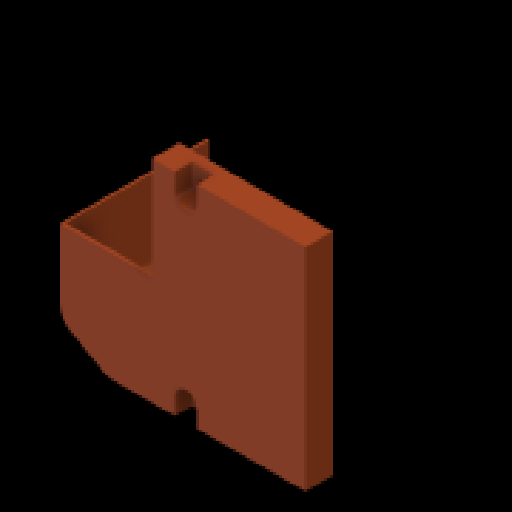
# Autodesk Inventor part: Extruder Cover
Saved by Autodesk Inventor 2023.3 (Build 273359000, 359)
## iProperties
Created: 2023-02-08
Part Number: Extruder Cover
Material: ABS Plastic
Document SubType Name: Modeling
Designer: remop
Density: 1.06 g/cm^3
Appearance: Smooth - Light Orange
Author: remop
Autodesk Inventor part; units mm, degrees
ref_plane "YZ Plane" through (0, 0, 0) normal (1, 0, 0) x (0, 1, 0)
ref_plane "XZ Plane" through (0, 0, 0) normal (0, 1, 0) x (-1, 0, 0)
ref_plane "XY Plane" through (0, 0, 0) normal (0, 0, 1) x (1, 0, 0)
sketch "Sketch1" plane through (0, 0, 0) normal (0, 0, 1) x (1, 0, 0)
  circle A0 centre (-5, 44) radius 1.4 projected
  circle A1 centre (-5, -8) radius 1.4 projected
  circle A2 centre (-5, 44) radius 1.75
  circle A3 centre (-5, -8) radius 1.75
  circle A4 centre (-5, -8) radius 3.25
  line L0 (-10, 49) -> (30, 49) projected
  line L1 (-10, -13) -> (30, -13) projected
  circle A5 centre (-5, 44) radius 3.25
  line L2 (-1.75, 44) -> (-1.75, 49)
  line L3 (-1.75, -8) -> (-1.75, -13)
  line L4 (-8.25, 44) -> (-8.25, 49)
  line L5 (-8.25, -8) -> (-8.25, -13)
  line L6 (-39, 42.6491) -> (-29.3923, 48.1962) projected
  arc A6 (-39, 42.6491) -> (-42, 37.453) centre (-36, 37.453) ccw projected
  line L7 (-42, -1.453) -> (-42, 37.453) projected
  arc A7 (-42, -1.453) -> (-39, -6.6491) centre (-36, -1.453) ccw projected
  line L8 (-39, -6.6491) -> (-29.3923, -12.1962) projected
  arc A8 (-29.3923, -12.1962) -> (-26.3923, -13) centre (-26.3923, -7) ccw projected
  line L9 (-26.3923, -13) -> (-21.4462, -13) projected
  arc A9 (-26.3923, 49) -> (-29.3923, 48.1962) centre (-26.3923, 43) ccw projected
  line L10 (-10, 49) -> (-38, 49) projected
  line L11 (-10, -13) -> (-21.4462, -13)
  line L12 (30, 49) -> (30, -13)
  circle A10 centre (-26.3923, -7) radius 6
  circle A11 centre (-36, -1.453) radius 6
  circle A12 centre (-36, 37.453) radius 6
  circle A13 centre (-26.3923, 43) radius 6
  line L13 (-29.3923, 48.1962) -> (-39, 42.6491)
  line L14 (-42, 37.453) -> (-42, -1.453)
  line L15 (-39, -6.6491) -> (-29.3923, -12.1962)
  line L16 (-26.3923, -13) -> (-8.25, -13)
  line L17 (-1.75, -13) -> (30, -13)
  line L18 (30, 49) -> (-1.75, 49)
  line L19 (-8.25, 49) -> (-26.3923, 49)
  point P0 (0, 0)
  dimension "d0" = 3.5
  dimension "d1" = 6.5
  constraints: 26 end point, 11 point on line, 8 coincident, 6 point on circle, 5 centre point, 5 tangent, 4 collinear, 4 vertical, 2 equal radius, 1 horizontal, 1 perpendicular, 1 vertical alignment, 11 other
  measures "d0" diameter of A3
  measures "d1" diameter of A4
extrude "Extrusion1" add sketch "Sketch1" along normal blind 7 contours A4 L5 L1 L11 L9 A10 A11 L7 A12 A13 L10 L0 L4 A5 L2 L12 L3 | A8 A10 A11 | L8 A11 A10 | A7 A11 A10 | A10 A11 | A13 A12 A9 | A13 A12 L6 | A6 A12 A13 | A12 A13
sketch "Sketch2" plane through (0, 0, 7) normal (0, 0, 1) x (1, 0, 0)
  line L0 (30, 49) -> (-1.75, 49) projected
  line L1 (-1.75, 49) -> (-1.75, 44) projected
  arc A0 (-8.25, 44) -> (-1.75, 44) centre (-5, 44) ccw projected
  line L2 (-8.25, 44) -> (-8.25, 49) projected
  line L3 (-8.25, 49) -> (-26.3923, 49) projected
  arc A1 (-26.3923, 49) -> (-29.3923, 48.1962) centre (-26.3923, 43) ccw projected
  line L4 (-29.3923, 48.1962) -> (-39, 42.6491) projected
  arc A2 (-39, 42.6491) -> (-42, 37.453) centre (-36, 37.453) ccw projected
  line L5 (-42, 37.453) -> (-42, -1.453) projected
  arc A3 (-42, -1.453) -> (-39, -6.6491) centre (-36, -1.453) ccw projected
  line L6 (-39, -6.6491) -> (-29.3923, -12.1962) projected
  arc A4 (-29.3923, -12.1962) -> (-26.3923, -13) centre (-26.3923, -7) ccw projected
  line L7 (-26.3923, -13) -> (-8.25, -13) projected
  line L8 (-8.25, -13) -> (-8.25, -8) projected
  arc A5 (-1.75, -8) -> (-8.25, -8) centre (-5, -8) ccw projected
  line L9 (-1.75, -8) -> (-1.75, -13) projected
  line L10 (-1.75, -13) -> (30, -13) projected
  line L11 (30, -13) -> (30, 49) projected
  line L12 (-0.95, 48.2) -> (29.2, 48.2)
  line L13 (29.2, 48.2) -> (29.2, -12.2)
  line L14 (29.2, -12.2) -> (-0.95, -12.2)
  line L15 (-0.95, -12.2) -> (-0.95, -8)
  arc A6 (-0.95, -8) -> (-9.05, -8) centre (-5, -8) ccw
  line L16 (-9.05, -8) -> (-9.05, -12.2)
  line L17 (-9.05, -12.2) -> (-26.3923, -12.2)
  arc A7 (-28.9923, -11.5033) -> (-26.3923, -12.2) centre (-26.3923, -7) ccw
  line L18 (-28.9923, -11.5033) -> (-38.6, -5.9563)
  arc A8 (-41.2, -1.453) -> (-38.6, -5.9563) centre (-36, -1.453) ccw
  line L19 (-41.2, -1.453) -> (-41.2, 37.453)
  arc A9 (-38.6, 41.9563) -> (-41.2, 37.453) centre (-36, 37.453) ccw
  line L20 (-38.6, 41.9563) -> (-28.9923, 47.5033)
  arc A10 (-26.3923, 48.2) -> (-28.9923, 47.5033) centre (-26.3923, 43) ccw
  line L21 (-26.3923, 48.2) -> (-9.05, 48.2)
  line L22 (-9.05, 48.2) -> (-9.05, 44)
  arc A11 (-9.05, 44) -> (-0.95, 44) centre (-5, 44) ccw
  line L23 (-0.95, 44) -> (-0.95, 48.2)
  point P0 (0, 0)
  dimension "d4" = 0.8
  constraints: 24 end point, 12 point on circle, 6 centre point, 17 other
  measures "d4" distance between parallel lines of L0 L12
extrude "Extrusion2" cut sketch "Sketch2" against normal through all contours L12 L13 L14 L15 A6 L16 L17 A7 L18 A8 L19 A9 L20 A10 L21 L22 A11 L23
sketch "Sketch3" plane through (0, 0, 7) normal (0, 0, 1) x (1, 0, 0)
  arc A0 (-38.6, 41.9563) -> (-41.2, 37.453) centre (-36, 37.453) ccw projected
  line L0 (-38.6, 41.9563) -> (-28.9923, 47.5033) projected
  arc A1 (-26.3923, 48.2) -> (-28.9923, 47.5033) centre (-26.3923, 43) ccw projected
  line L1 (-26.3923, 48.2) -> (-9.05, 48.2) projected
  line L2 (-9.05, 48.2) -> (-9.05, 44) projected
  arc A2 (-9.05, 44) -> (-0.95, 44) centre (-5, 44) ccw projected
  line L3 (-0.95, 44) -> (-0.95, 48.2) projected
  line L4 (-0.95, 48.2) -> (29.2, 48.2) projected
  line L5 (29.2, 48.2) -> (29.2, -12.2) projected
  line L6 (29.2, -12.2) -> (-0.95, -12.2) projected
  line L7 (-0.95, -12.2) -> (-0.95, -8) projected
  arc A3 (-0.95, -8) -> (-9.05, -8) centre (-5, -8) ccw projected
  line L8 (-9.05, -8) -> (-9.05, -12.2) projected
  line L9 (-9.05, -12.2) -> (-26.3923, -12.2) projected
  arc A4 (-28.9923, -11.5033) -> (-26.3923, -12.2) centre (-26.3923, -7) ccw projected
  line L10 (-28.9923, -11.5033) -> (-38.6, -5.9563) projected
  arc A5 (-41.2, -1.453) -> (-38.6, -5.9563) centre (-36, -1.453) ccw projected
  line L11 (-41.2, -1.453) -> (-41.2, 37.453) projected
  line L12 (30, 49) -> (-1.75, 49) projected
  line L13 (-1.75, 49) -> (-1.75, 44) projected
  arc A6 (-8.25, 44) -> (-1.75, 44) centre (-5, 44) ccw projected
  line L14 (-8.25, 44) -> (-8.25, 49) projected
  line L15 (-8.25, 49) -> (-26.3923, 49) projected
  arc A7 (-26.3923, 49) -> (-29.3923, 48.1962) centre (-26.3923, 43) ccw projected
  line L16 (-29.3923, 48.1962) -> (-39, 42.6491) projected
  arc A8 (-39, 42.6491) -> (-42, 37.453) centre (-36, 37.453) ccw projected
  line L17 (-42, 37.453) -> (-42, -1.453) projected
  arc A9 (-42, -1.453) -> (-39, -6.6491) centre (-36, -1.453) ccw projected
  line L18 (-39, -6.6491) -> (-29.3923, -12.1962) projected
  arc A10 (-29.3923, -12.1962) -> (-26.3923, -13) centre (-26.3923, -7) ccw projected
  line L19 (-26.3923, -13) -> (-8.25, -13) projected
  line L20 (-8.25, -13) -> (-8.25, -8) projected
  arc A11 (-1.75, -8) -> (-8.25, -8) centre (-5, -8) ccw projected
  line L21 (-1.75, -8) -> (-1.75, -13) projected
  line L22 (-1.75, -13) -> (30, -13) projected
  line L23 (30, -13) -> (30, 49) projected
  point P0 (0, 0)
extrude "Extrusion3" add sketch "Sketch3" along normal blind 1 contours L0 A1 L1 L2 A2 L3 L4 L5 L6 L7 A3 L8 L9 A4 L10 A5 L11 A0 | L23 L22 L21 A11 L20 L19 A10 L18 A9 L17 A8 L16 A7 L15 L14 A6 L13 L12
sketch "Sketch4" plane through (0, 0, 8) normal (0, 0, 1) x (1, 0, 0)
  line L0 (-1.75, -13) -> (30, -13) projected
  line L1 (30, -13) -> (30, 49) projected
  line L2 (30, 49) -> (-1.75, 49) projected
  line L3 (-1.75, 49) -> (-1.75, 44) projected
  arc A0 (-8.25, 44) -> (-1.75, 44) centre (-5, 44) ccw projected
  line L4 (-8.25, 44) -> (-8.25, 49) projected
  line L5 (-8.25, 49) -> (-26.3923, 49) projected
  arc A1 (-26.3923, 49) -> (-29.3923, 48.1962) centre (-26.3923, 43) ccw projected
  line L6 (-29.3923, 48.1962) -> (-39, 42.6491) projected
  arc A2 (-39, 42.6491) -> (-42, 37.453) centre (-36, 37.453) ccw projected
  line L7 (-42, 37.453) -> (-42, -1.453) projected
  arc A3 (-42, -1.453) -> (-39, -6.6491) centre (-36, -1.453) ccw projected
  line L8 (-39, -6.6491) -> (-29.3923, -12.1962) projected
  arc A4 (-29.3923, -12.1962) -> (-26.3923, -13) centre (-26.3923, -7) ccw projected
  line L9 (-26.3923, -13) -> (-8.25, -13) projected
  line L10 (-8.25, -13) -> (-8.25, -8) projected
  arc A5 (-1.75, -8) -> (-8.25, -8) centre (-5, -8) ccw projected
  line L11 (-1.75, -8) -> (-1.75, -13) projected
  line L12 (-8.25, 49) -> (-26.3923, 49) projected
  line L13 (-15, 49) -> (-15, 19)
  line L14 (-15, 19) -> (-42, 19)
  point P0 (0, 0)
  dimension "d9" = 30
  dimension "d10" = 27
  constraints: 4 end point, 2 point on line, 1 perpendicular, 1 vertical
  measures "d9" distance of L13.start L13.end
  measures "d10" distance of L13.end L14.end
extrude "Extrusion4" cut sketch "Sketch4" against normal through all contours L13 L14 L7 A2 L6 A1 L5
sketch "Sketch5" plane through (0, 0, 0) normal (0, 0, -1) x (-1, 0, 0)
  line L0 (15, 48.2) -> (15, 49) projected
  line L1 (8.25, 49) -> (15, 49) projected
  line L2 (8.25, 44) -> (8.25, 49) projected
  arc A0 (1.75, 44) -> (8.25, 44) centre (5, 44) ccw projected
  line L3 (1.75, 49) -> (1.75, 44) projected
  line L4 (-30, 49) -> (1.75, 49) projected
  line L5 (-30, -13) -> (-30, 49) projected
  line L6 (1.75, -13) -> (-30, -13) projected
  line L7 (1.75, -8) -> (1.75, -13) projected
  arc A1 (8.25, -8) -> (1.75, -8) centre (5, -8) ccw projected
  line L8 (8.25, -13) -> (8.25, -8) projected
  line L9 (26.3923, -13) -> (8.25, -13) projected
  arc A2 (26.3923, -13) -> (29.3923, -12.1962) centre (26.3923, -7) ccw projected
  line L10 (39, -6.6491) -> (29.3923, -12.1962) projected
  arc A3 (39, -6.6491) -> (42, -1.453) centre (36, -1.453) ccw projected
  line L11 (42, 19) -> (42, -1.453) projected
  line L12 (42, 19) -> (41.2, 19) projected
  line L13 (41.2, 19) -> (41.2, -1.453) projected
  arc A4 (38.6, -5.9563) -> (41.2, -1.453) centre (36, -1.453) ccw projected
  line L14 (38.6, -5.9563) -> (28.9923, -11.5033) projected
  arc A5 (26.3923, -12.2) -> (28.9923, -11.5033) centre (26.3923, -7) ccw projected
  line L15 (26.3923, -12.2) -> (9.05, -12.2) projected
  line L16 (9.05, -12.2) -> (9.05, -8) projected
  arc A6 (9.05, -8) -> (0.95, -8) centre (5, -8) ccw projected
  line L17 (0.95, -8) -> (0.95, -12.2) projected
  line L18 (0.95, -12.2) -> (-29.2, -12.2) projected
  line L19 (-29.2, -12.2) -> (-29.2, 48.2) projected
  line L20 (-29.2, 48.2) -> (0.95, 48.2) projected
  line L21 (0.95, 48.2) -> (0.95, 44) projected
  arc A7 (0.95, 44) -> (9.05, 44) centre (5, 44) ccw projected
  line L22 (9.05, 44) -> (9.05, 48.2) projected
  line L23 (9.05, 48.2) -> (15, 48.2) projected
  line L24 (10, -13) -> (10, 49) projected
  point P0 (0, 0)
  point P1 (10, -12.2)
extrude "Extrusion5" add sketch "Sketch5" along normal blind 35 contours L15 A5 L14 A4 L13 L12 L11 A3 L10 A2 L9 L24
sketch "Sketch6" plane through (0, 0, 0) normal (0, 0, -1) x (-1, 0, 0)
  arc A0 (8.25, -8) -> (1.75, -8) centre (5, -8) ccw projected
  arc A1 (1.75, 44) -> (8.25, 44) centre (5, 44) ccw projected
  line L0 (10, -13) -> (-30, -13) projected
  line L1 (1.75, -8) -> (1.75, -13) projected
  line L2 (1.75, -8) -> (1.75, -13)
  line L3 (1.75, -13) -> (8.25, -13)
  line L4 (8.25, -13) -> (8.25, -8)
  line L5 (26.3923, 49) -> (-4, 49) projected
  line L6 (1.75, 49) -> (1.75, 44) projected
  line L7 (1.75, 44) -> (1.75, 49)
  line L8 (8.25, 44) -> (8.25, 49) projected
  line L9 (1.75, 49) -> (8.25, 49)
  line L10 (8.25, 49) -> (8.25, 44)
  circle A2 centre (5, 44) radius 1.75
  circle A3 centre (5, -8) radius 1.75
  point P0 (0, 0)
  dimension "d15" = 3.5
  constraints: 12 end point, 2 centre point, 2 coincident, 2 collinear, 2 perpendicular, 1 equal radius, 1 point on circle, 1 tangent, 1 vertical
  measures "d15" diameter of A2
extrude "Extrusion6" add sketch "Sketch6" against normal blind 3
body "Solid1"
